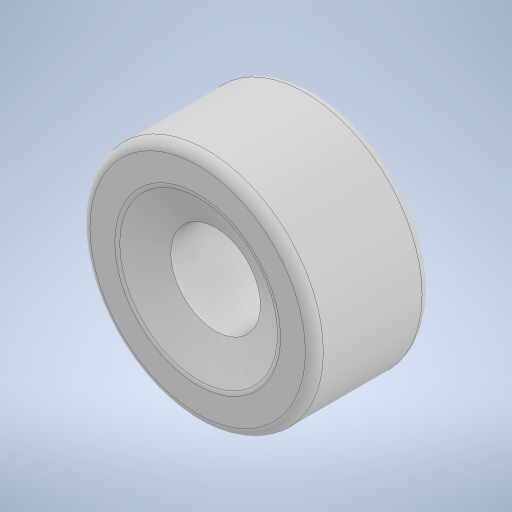
# Autodesk Inventor part: Wheel
Saved by Autodesk Inventor 2023 (Build 270158000, 158)
## iProperties
Created: 2024-03-04
Part Number: Wheel
Material: Generic
Document SubType Name: Modeling
Designer: pavel
Density: 1 g/cm^3
Appearance: Default
Author: pavel
Autodesk Inventor part; units mm, degrees
ref_plane "YZ Plane" through (0, 0, 0) normal (1, 0, 0) x (0, 1, 0)
ref_plane "XZ Plane" through (0, 0, 0) normal (0, 1, 0) x (-1, 0, 0)
ref_plane "XY Plane" through (0, 0, 0) normal (0, 0, 1) x (1, 0, 0)
sketch "Sketch1" plane through (0, 0, 0) normal (0, 0, 1) x (1, 0, 0)
  circle A0 centre (0, 0) radius 13
  dimension "d0" = 26
  constraints: 1 centre point, 1 coincident
  measures "d0" diameter of A0
extrude "Extrusion1" add sketch "Sketch1" along normal blind 13
sketch "Sketch2" plane through (0, 0, 13) normal (0, 0, 1) x (1, 0, 0)
  circle A0 centre (0, 0) radius 13 projected
  constraints: 1 coincident
hole "Hole1" at (0, 0, 13) direction (0, 0, -1) diameter 10 end through all
sketch "Sketch3" plane through (0, 0, 0) normal (0, 1, 0) x (-1, 0, 0)
  line L0 (0, 13) -> (0, 0)
  line L1 (-5, 13) -> (5, 13) projected
  line L2 (13, 13) -> (-13, 13) projected
  line L3 (5, 0) -> (5, 13) projected
  line L4 (5, 11) -> (9, 13)
  line L5 (9, 13) -> (5, 13)
  line L6 (5, 13) -> (5, 11)
  dimension "d10" = 2
  dimension "d11" = 4
  constraints: 8 end point, 2 collinear, 2 point on line, 1 coincident, 1 midpoint, 1 vertical
  measures "d10" distance of L1.end L4.start
  measures "d11" horizontal distance of L4.end L4.start
revolve "Revolution1" cut sketch "Sketch3" angle 360 about axis through (0, 0, 13) along (0, 0, -1)
ref_plane "Work Plane1" through (0, 0, 6.5) normal (0, 0, 1) x (1, 0, 0)
mirror "Mirror1" about plane through (0, 0, 6.5) normal (0, 0, 1) of "Revolution1"
fillet "Fillet1" radius 1 4 edges at (-13, 0, 0) (9, 0, 0) (-13, 0, 13) (9, 0, 13)
body "Solid1"
